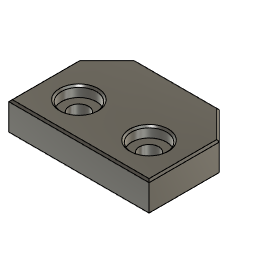
fixated locating tabs (Autodesk Fusion 360 design; units mm, degrees)
Autodesk Fusion 360 part; units mm, degrees
sketch "Sketch1" plane through (0, 0, 0) normal (0, 0, 1) x (1, 0, 0)
  line L0 (0, 0) -> (40, 0)
  line L1 (40, 0) -> (40, 28)
  line L2 (40, 28) -> (0, 28)
  line L3 (0, 28) -> (0, 0)
  line L4 (0, 0) -> (40, 0) construction
  line L5 (40, 0) -> (40, 20) construction
  line L6 (40, 20) -> (0, 20) construction
  line L7 (0, 20) -> (0, 0) construction
  line L8 (0, 20) -> (20, 20) construction
  line L9 (20, 20) -> (20, 0) construction
  line L10 (20, 0) -> (0, 0) construction
  line L11 (0, 0) -> (0, 20) construction
  line L12 (0, 0) -> (20, 20) construction
  line L13 (0, 20) -> (20, 0) construction
  line L14 (20, 20) -> (40, 0) construction
  line L15 (20, 0) -> (40, 20) construction
  circle A0 centre (10, 10) radius 5
  circle A1 centre (30, 10) radius 5
  dimension "d1" = 40
  dimension "d2" = 28
  dimension "d3" = 20
  dimension "d4" = 10
  dimension "d5" = 10
  constraint horizontal L0
  constraint vertical L1
  constraint horizontal L2
  constraint vertical L3
  constraint coincident L0.start L3.end
  constraint horizontal L4
  constraint vertical L5
  constraint horizontal L6
  constraint vertical L7
  constraint horizontal L8
  constraint vertical L9
  constraint horizontal L10
  constraint vertical L11
  constraint midpoint L4 L9.end
  constraint perpendicular L12 L13
  constraint midpoint L12 A0.centre
  constraint midpoint L14 A1.centre
  measures "d1" distance of L0.start L0.end
  measures "d2" distance of L0.start L2.end
  measures "d3" distance of L0.start L6.end
  measures "d4" diameter of A0
  measures "d5" diameter of A1
extrude "Extrude1" add sketch "Sketch1" against normal blind 3
sketch "Sketch2" plane through (0, 0, -3) normal (0, 0, -1) x (1, 0, 0)
  circle A0 centre (10, -10) radius 5
  circle A1 centre (30, -10) radius 5
  line L0 (0, 0) -> (0, -28)
  line L1 (0, -28) -> (40, -28)
  line L2 (40, -28) -> (40, 0)
  line L3 (40, 0) -> (0, 0)
  circle A2 centre (30, -10) radius 2.75
  circle A3 centre (10, -10) radius 2.75
  dimension "d8" = 5.5
  dimension "d9" = 5.5
  constraint concentric A1 A2
  constraint concentric A0 A3
  measures "d8" diameter of A2
  measures "d9" diameter of A3
extrude "Extrude2" add sketch "Sketch2" along normal blind 5 contours A0 | A1 | L0 L1 L2 L3
chamfer "Chamfer1" distance 8 angle 45 1 edges at (0, 28, -4)
chamfer "Chamfer2" distance 8 angle 45 1 edges at (40, 28, -4)
chamfer "Chamfer3" distance 0.5 angle 45 8 edges at (4, 24, 0) (0, 10, 0) (20, 0, 0) (40, 10, 0) (36, 24, 0) (20, 28, 0) (5.3384, 11.8081, 0) (25.3384, 11.8081, 0)
